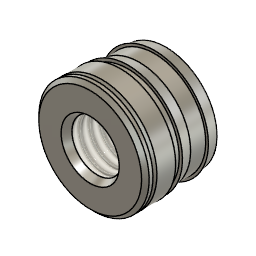
Hackpad (Autodesk Fusion 360 archive; units mm, degrees)
design "Tapered Open End Insert - M3 X 3.81 Stainless Steel Plain"
description: Tapered Open End Insert - M3 X 3.81
part number: TOEI - M3 X 3.81 Stainless Steel Plain
Autodesk Fusion 360 part; units mm, degrees
sketch "Sketch2" plane through (0, 0, 0) normal (1, 0, 0) x (0, 1, 0)
  line L0 (0, -3.81) -> (0, 0)
  line L1 (1.5, -3.81) -> (1.5, 0)
  line L2 (1.5, 0) -> (2.5895, 0)
  line L3 (2.5895, 0) -> (2.78, -0.1905)
  line L4 (2.78, -0.1905) -> (2.78, -0.381)
  line L5 (2.78, -0.381) -> (2.58, -0.381)
  line L6 (2.58, -0.381) -> (2.78, -0.581)
  line L7 (2.78, -0.581) -> (2.78, -1.524)
  line L8 (2.78, -1.524) -> (2.58, -1.524)
  line L9 (2.58, -1.524) -> (2.58, -1.905)
  line L10 (2.58, -1.905) -> (2.74, -1.905)
  line L11 (2.74, -1.905) -> (2.58, -2.4765)
  line L12 (2.58, -2.4765) -> (2.58, -3.2385)
  line L13 (2.7133, -3.2385) -> (2.58, -3.81)
  line L14 (2.58, -3.81) -> (1.5, -3.81)
  line L15 (2.58, -3.2385) -> (2.7133, -3.2385)
  point P0 (1.5, 0)
  dimension "d48" = 5.56
  dimension "d50" = 5.16
  dimension "d51" = 1.905
  dimension "d52" = 45
  dimension "d53" = 1.524
  dimension "d54" = 0.381
  dimension "d55" = 45
  dimension "d57" = 5.48
  dimension "d58" = 5.4267
  dimension "d61" = 3
  dimension "d81" = 3.81
  dimension "d96" = 0.5715
  dimension "d98" = 0.1905
  dimension "d99" = 0.5715
  constraint vertical L1
  constraint collinear L4 L7
  constraint coincident L12 L13.end
  constraint collinear L9 L12
  constraint vertical L5.end L8.end
  constraint coincident P0 L1
  constraint coincident P0 L2
  constraint coincident L0.end origin
  constraint coincident L0.start L14
  constraint coincident L0.end L2
  constraint horizontal L14
  constraint perpendicular L9 L10
  constraint coincident P0 L1.end
  measures "d51" distance of L10 L14
  measures "d52" angle of L5 L6
  measures "d53" distance of L2 L8
  measures "d54" distance of L2 L5
  measures "d55" angle of L2 L3
  measures "d81" distance of L2 L14
  measures "d96" distance of L10 L11.end
  measures "d98" distance of L2.end L4
  measures "d99" distance of L14 L15
revolve "Revolve2" add sketch "Sketch2" angle 360 about axis through (0, 0, -3.81) along (0, 0, 1)
thread "Thread4" "ISO Metric profile 3.0 M3x0.5 M3x0.5 6H" major diameter 3.086 minor diameter 2.529 pitch 0.5 angle 60 resizes the face on face at (0.1494, 1.4925, -2.54)
chamfer "Chamfer2" distance 0.2 angle 60 2 edges at (-0.4573, -1.1789, 0) (-0.4573, -1.1789, -3.81) measured on face at (-0.1915, 2.1335, 0) measured on face at (0.1259, 1.2582, -2.54)
equation "d48 = adsk_maxdia"
equation "d50 = adsk_leaddia"
equation "d51 = adsk_nheig * 0.5"
equation "d53 = adsk_nheig * 0.4"
equation "d54 = adsk_nheig * 0.1"
equation "d57 = adsk_maxdia - ( adsk_maxdia - adsk_leaddia ) / 5"
equation "d58 = adsk_maxdia - ( adsk_maxdia - adsk_leaddia ) / 3"
equation "d61 = adsk_nomdia"
equation "d81 = adsk_nheig"
equation "adsk_nheig = 3.81 mm"
equation "adsk_maxdia = 5.56 mm"
equation "adsk_leaddia = 5.16 mm"
equation "adsk_nomdia = 3.00 mm"
equation "d96 = adsk_nheig * 0.5 * 0.3"
equation "d98 = adsk_nheig * 0.1 / 2"
equation "d99 = adsk_nheig * 0.5 * 0.3"
